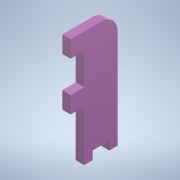
# Autodesk Inventor part: Side
Saved by Autodesk Inventor 2022 (Build 260153000, 153)
## iProperties
Created: 2021-07-09
Part Number: Side
Material: Generic
Document SubType Name: Modeling
Designer: benka
Density: 1 g/cm^3
Appearance: Smooth - Purple
Author: benka
Autodesk Inventor part; units mm, degrees
ref_plane "YZ Plane" through (0, 0, 0) normal (1, 0, 0) x (0, 1, 0)
ref_plane "XZ Plane" through (0, 0, 0) normal (0, 1, 0) x (-1, 0, 0)
ref_plane "XY Plane" through (0, 0, 0) normal (0, 0, 1) x (1, 0, 0)
sketch "dds" plane through (0, -35.5355, 2.0355) normal (1, 0, 0) x (0, 1, 0)
  line L0 (0, -9.9999) -> (5, -9.9999)
  line L1 (0, -9.9999) -> (0, -15)
  line L2 (0, -15) -> (5, -15)
  line L3 (0, 0) -> (5, 0)
  line L4 (5, -9.9999) -> (5, 0)
  line L5 (5, -15) -> (59, -15)
  line L6 (0, 0) -> (0, 5)
  line L7 (69, 5) -> (69, 13)
  line L8 (69, 5) -> (69, -5)
  arc A0 (59, -15) -> (69, -5) centre (59, -5) ccw
  line L9 (69, 13) -> (58.8965, 13)
  line L10 (58.8965, 13) -> (58.8965, 5)
  line L11 (40.1783, 13) -> (30.0747, 13)
  line L12 (40.1783, 5) -> (40.1783, 13)
  line L13 (30.0747, 13) -> (30.0747, 5)
  line L14 (0, 5) -> (30.0747, 5)
  line L15 (40.1783, 5) -> (58.8965, 5)
  point P0 (69, -15)
  point P1 (8.1162, -2.0146)
  dimension "d0" = 10
  dimension "d1" = 8
  constraints: 32 end point, 4 perpendicular, 3 horizontal, 3 vertical, 2 collinear, 2 point on circle, 2 point on line, 2 tangent, 1 centre point
  measures "d0" radius of A0
  measures "d1" distance of L7.start L7.end
extrude "Side" add sketch "dds" along normal blind 5
body "Solid1"
